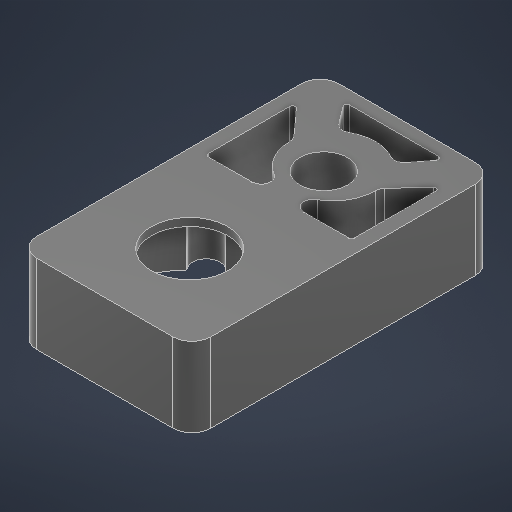
# Autodesk Inventor part: CapOGStyle
Saved by Autodesk Inventor 2026.1 (Build 301233000, 233)
## iProperties
Created: 2023-06-22
Part Number: CapOGStyle
Material: Plastic, Opaque Black
Document SubType Name: Modeling
Designer: Teddy
Density: 0.952 g/cm^3
Appearance: Smooth - Black
Author: Teddy
Autodesk Inventor part; units mm, degrees
ref_plane "YZ Plane" through (0, 0, 0) normal (1, 0, 0) x (0, 1, 0)
ref_plane "XZ Plane" through (0, 0, 0) normal (0, 1, 0) x (-1, 0, 0)
ref_plane "XY Plane" through (0, 0, 0) normal (0, 0, 1) x (1, 0, 0)
sketch "Sketch5" plane through (0, 0, 0) normal (0, 1, 0) x (-1, 0, 0)
  line L0 (-12.8932, 28.65) -> (12.9, 28.65)
  line L1 (16.5, 25.05) -> (16.5, -25.0432)
  line L2 (12.8932, -28.65) -> (-12.8932, -28.65)
  line L3 (-16.5, -25.0432) -> (-16.5, 25.0432)
  line L4 (-16.5, 28.65) -> (16.5, -28.65) construction
  line L5 (16.5, 28.65) -> (-16.5, -28.65) construction
  arc A0 (16.5, 25.05) -> (12.9, 28.65) centre (12.9, 25.05) ccw
  line L6 (12.9, 28.65) -> (12.9, 25.05) construction
  line L7 (12.9, 25.05) -> (16.5, 25.05) construction
  arc A1 (12.8932, -28.65) -> (16.5, -25.0432) centre (12.8932, -25.0432) ccw
  arc A2 (-12.8932, 28.65) -> (-16.5, 25.0432) centre (-12.8932, 25.0432) ccw
  arc A3 (-16.5, -25.0432) -> (-12.8932, -28.65) centre (-12.8932, -25.0432) ccw
  circle A4 centre (13.5, 25.6528) radius 0.9915
  line L8 (11.2085, 27.55) -> (-11.2085, 27.55)
  arc A5 (-15.517, 25.05) -> (-15.517, 25.0432) centre (-12.8932, 25.0432) ccw
  line L9 (-15.4, 23.3613) -> (-15.4, -23.3613)
  line L10 (-11.2085, -27.55) -> (11.2085, -27.55)
  line L11 (15.4, -23.3613) -> (15.4, 23.3613)
  line L12 (12.5085, 25.6528) -> (12.5085, 26.25)
  line L13 (13.5, 24.6613) -> (14.1, 24.6613)
  arc A6 (12.5085, 26.25) -> (11.2085, 27.55) centre (11.2085, 26.25) ccw
  arc A7 (15.4, 23.3613) -> (14.1, 24.6613) centre (14.1, 23.3613) ccw
  line L14 (15.4, 0) -> (-15.4, 0) construction
  line L15 (0, 27.55) -> (0, -27.55) construction
  circle A8 centre (13.5, -25.6528) radius 0.9915
  line L16 (12.5085, -25.6528) -> (12.5085, -26.25)
  line L17 (13.5, -24.6613) -> (14.1, -24.6613)
  arc A9 (11.2085, -27.55) -> (12.5085, -26.25) centre (11.2085, -26.25) ccw
  arc A10 (14.1, -24.6613) -> (15.4, -23.3613) centre (14.1, -23.3613) ccw
  line L18 (0, -27.55) -> (0, 27.55) construction
  circle A11 centre (-13.5, 25.6528) radius 0.9915
  line L19 (-12.5085, 25.6528) -> (-12.5085, 26.25)
  line L20 (-13.5, 24.6613) -> (-14.1, 24.6613)
  arc A12 (-11.2085, 27.55) -> (-12.5085, 26.25) centre (-11.2085, 26.25) ccw
  arc A13 (-14.1, 24.6613) -> (-15.4, 23.3613) centre (-14.1, 23.3613) ccw
  arc A14 (-12.5085, -26.25) -> (-11.2085, -27.55) centre (-11.2085, -26.25) ccw
  line L21 (-12.5085, -25.6528) -> (-12.5085, -26.25)
  circle A15 centre (-13.5, -25.6528) radius 0.9915
  line L22 (-13.5, -24.6613) -> (-14.1, -24.6613)
  arc A16 (-15.4, -23.3613) -> (-14.1, -24.6613) centre (-14.1, -23.3613) ccw
  line L23 (-12.1355, -25.3386) -> (-12.1355, -25.333)
  line L24 (14.7139, 22.2154) -> (14.827, 22.0092) construction
  circle A17 centre (0, 12.583) radius 7.25
  arc A18 (6.3593, 25.2794) -> (-6.3593, 25.2794) centre (0, 12.583) ccw
  arc A19 (-6.3593, -0.1134) -> (6.3593, -0.1134) centre (0, 12.583) ccw
  line L25 (0, 12.583) -> (-6.3593, -0.1134) construction
  line L26 (0, 12.583) -> (6.3593, -0.1134) construction
  line L27 (0, 12.583) -> (0, -1.617) construction
  line L28 (0, 12.583) -> (16.5, 12.583) construction
  line L29 (-6.3593, -0.1134) -> (-6.3593, 25.2794) construction
  line L30 (6.3593, -0.1134) -> (6.3593, 25.2794) construction
  arc A20 (-6.3593, -0.1134) -> (-6.9877, -0.2666) centre (-6.5832, -0.5605) ccw
  line L31 (-6.9877, -0.2666) -> (-6.5832, -0.5605) construction
  line L32 (-6.5832, -0.5605) -> (-6.3593, -0.1134) construction
  line L33 (-6.9877, -0.2666) -> (-7.2816, -0.671)
  arc A21 (-10.5175, 1.6804) -> (-7.2816, -0.671) centre (-8.8995, 0.5047) ccw
  line L34 (-10.5175, 1.6804) -> (-10.2236, 2.0849)
  arc A22 (-10.2236, 2.0849) -> (-10.2728, 2.7402) centre (-10.6345, 2.3835) ccw
  line L35 (-10.2236, 2.0849) -> (-10.6345, 2.3835) construction
  line L36 (-10.6345, 2.3835) -> (-10.2728, 2.7402) construction
  arc A23 (6.9877, -0.2666) -> (6.3593, -0.1134) centre (6.5832, -0.5605) ccw
  line L37 (6.9877, -0.2666) -> (7.2816, -0.671)
  arc A24 (7.2816, -0.671) -> (10.5175, 1.6804) centre (8.8995, 0.5047) ccw
  line L38 (10.5175, 1.6804) -> (10.2236, 2.0849)
  arc A25 (10.2728, 2.7402) -> (10.2236, 2.0849) centre (10.6345, 2.3835) ccw
  arc A26 (-6.9877, 25.4326) -> (-6.3593, 25.2794) centre (-6.5832, 25.7265) ccw
  line L39 (-6.9877, 25.4326) -> (-7.2816, 25.837)
  arc A27 (-7.2816, 25.837) -> (-10.5175, 23.4856) centre (-8.8995, 24.6613) ccw
  line L40 (-10.5175, 23.4856) -> (-10.2236, 23.0811)
  arc A28 (-10.2728, 22.4258) -> (-10.2236, 23.0811) centre (-10.6345, 22.7825) ccw
  arc A29 (6.3593, 25.2794) -> (6.9877, 25.4326) centre (6.5832, 25.7265) ccw
  line L41 (6.9877, 25.4326) -> (7.2816, 25.837)
  arc A30 (10.5175, 23.4856) -> (7.2816, 25.837) centre (8.8995, 24.6613) ccw
  line L42 (10.5175, 23.4856) -> (10.2236, 23.0811)
  arc A31 (10.2236, 23.0811) -> (10.2728, 22.4258) centre (10.6345, 22.7825) ccw
  arc A32 (-10.2728, 22.4258) -> (-10.2728, 2.7402) centre (0, 12.583) ccw
  arc A33 (10.2728, 2.7402) -> (10.2728, 22.4258) centre (0, 12.583) ccw
  circle A34 centre (0, -12.96) radius 3.955
  line L43 (0, -12.96) -> (0, -18.96) construction
  circle A35 centre (13.5, -25.6528) radius 2
  line L44 (13.5, -25.6528) -> (13.5, -23.6528) construction
  line L45 (13.5, -25.6528) -> (11.5, -25.6528) construction
  line L46 (13.5, -23.6528) -> (15.3669, -23.6528) construction
  line L47 (11.5, -25.6528) -> (11.5, -27.5169) construction
  circle A36 centre (-13.5, -25.6528) radius 2
  circle A37 centre (-13.5, 25.6528) radius 2
  circle A38 centre (13.5, 25.6528) radius 2
  circle A39 centre (0, -12.843) radius 4.5212
  circle A40 centre (0, -14.56) radius 6.25
  line L48 (0, -14.56) -> (-5.807, -24.618) construction
  line L49 (0, -14.56) -> (5.807, -24.618) construction
  arc A41 (-4.057, -21.5869) -> (4.057, -21.5869) centre (0, -14.56) ccw
  arc A42 (-4.057, -21.5869) -> (-6.3593, -22.0899) centre (-4.932, -23.1025) ccw
  arc A43 (6.3306, -22.0506) -> (4.057, -21.5869) centre (4.932, -23.1025) ccw
  line L50 (0, -26.174) -> (-8.43, -26.174)
  line L51 (0, -26.174) -> (8.4301, -26.174)
  line L52 (8.8297, -25.3735) -> (6.3306, -22.0506)
  arc A44 (8.4301, -26.174) -> (8.8297, -25.3735) centre (8.4301, -25.674) ccw
  line L53 (-8.8295, -25.3734) -> (-6.3593, -22.0899)
  arc A45 (-8.8295, -25.3734) -> (-8.43, -26.174) centre (-8.43, -25.674) ccw
  line L54 (-4.8269, -4.2707) -> (-13.3585, -4.2707)
  line L55 (-13.8585, -4.7707) -> (-13.8585, -20.2911)
  line L56 (-12.9875, -20.6263) -> (-8.5656, -15.7334)
  arc A46 (-13.8585, -20.2911) -> (-12.9875, -20.6263) centre (-13.3585, -20.2911) ccw
  arc A47 (-13.3585, -4.2707) -> (-13.8585, -4.7707) centre (-13.3585, -4.7707) ccw
  line L57 (5.0371, -4.2707) -> (13.3585, -4.2707)
  line L58 (13.8585, -4.7707) -> (13.8585, -20.2921)
  line L59 (12.9875, -20.6273) -> (8.5655, -15.7332)
  arc A48 (12.9875, -20.6273) -> (13.8585, -20.2921) centre (13.3585, -20.2921) ccw
  arc A49 (13.8585, -4.7707) -> (13.3585, -4.2707) centre (13.3585, -4.7707) ccw
  arc A50 (8.114, -14.56) -> (4.057, -7.5331) centre (0, -14.56) ccw
  arc A51 (-4.057, -7.5331) -> (-8.114, -14.56) centre (0, -14.56) ccw
  arc A52 (8.114, -14.56) -> (8.5655, -15.7332) centre (9.864, -14.56) ccw
  arc A53 (5.0371, -4.2707) -> (4.057, -7.5331) centre (5.0371, -6.0491) ccw
  arc A54 (-4.057, -7.5331) -> (-4.8269, -4.2707) centre (-4.8269, -5.9927) ccw
  arc A55 (-8.5656, -15.7334) -> (-8.114, -14.56) centre (-9.864, -14.56) ccw
  line L60 (10.7841, 22.7925) -> (11.0216, 23.1193)
  arc A56 (11.0216, 23.1193) -> (6.7775, 26.2034) centre (8.8995, 24.6613) ccw
  line L61 (6.7775, 26.2034) -> (6.5448, 25.883)
  arc A57 (6.5448, 25.883) -> (-6.5448, 25.883) centre (0, 12.583) ccw
  line L62 (-6.5448, 25.883) -> (-6.7775, 26.2034)
  arc A58 (-6.7775, 26.2034) -> (-11.0216, 23.1193) centre (-8.8995, 24.6613) ccw
  line L63 (-11.0216, 23.1193) -> (-10.7841, 22.7925)
  arc A59 (-10.7841, 22.7925) -> (-10.7841, 2.3735) centre (0, 12.583) ccw
  line L64 (-10.7841, 2.3735) -> (-11.0216, 2.0467)
  arc A60 (-11.0216, 2.0467) -> (-6.7775, -1.0374) centre (-8.8995, 0.5047) ccw
  line L65 (-6.7775, -1.0374) -> (-6.5448, -0.717)
  arc A61 (-6.5448, -0.717) -> (6.5448, -0.717) centre (0, 12.583) ccw
  line L66 (6.5448, -0.717) -> (6.7775, -1.0374)
  arc A62 (6.7775, -1.0374) -> (11.0216, 2.0467) centre (8.8995, 0.5047) ccw
  line L67 (11.0216, 2.0467) -> (10.7841, 2.3735)
  arc A63 (10.7841, 2.3735) -> (10.7841, 22.7925) centre (0, 12.583) ccw
  point P0 (0, 0)
  point P1 (0, 0)
  point P2 (-2.4, 0)
  point P3 (-12.1591, 27.1367)
  point P4 (-14.9852, 24.3133)
  point P5 (-14.9852, -24.3133)
  point P6 (-12.1591, -27.1367)
  point P7 (12.1591, -27.1367)
  point P8 (14.9852, -24.3133)
  point P9 (14.9852, 24.3133)
  point P10 (12.1591, 27.1367)
  point P11 (5.807, -24.501)
  point P12 (13.8585, -4.2707)
  dimension "d61" = 57.3
  dimension "d62" = 33
  dimension "d63" = 3.6
  dimension "d64" = 90
  dimension "d65" = 3.6068
  dimension "d66" = 3.6068
  dimension "d67" = 2.9972
  dimension "d68" = 3
  dimension "d69" = 1.983
  dimension "d70" = 1.1
  dimension "d71" = 1.3
  dimension "d74" = 22.417
  dimension "d84" = 14.5
  dimension "d85" = 28.4
  dimension "d87" = 53.21
  dimension "d88" = 0.5
  dimension "d89" = 80.6
  dimension "d90" = 0.5
  dimension "d91" = 2
  dimension "d92" = 0.508
  dimension "d93" = 80.6
  dimension "d98" = 25.543
  dimension "d99" = 7.91
  dimension "d116" = 4
  dimension "d117" = 4
  dimension "d118" = 4
  dimension "d119" = 4
  dimension "d128" = 9.0424
  dimension "d129" = 1.6
  dimension "d130" = 12.5
  dimension "d131" = 60
  dimension "d132" = 30
  dimension "d145" = 0.5
  dimension "d146" = 0.5
  dimension "d147" = 0.5
  dimension "d148" = 0.5
  dimension "d151" = 360
  dimension "d192" = 1.1
  dimension "d193" = 1.1
  dimension "d195" = 1.1
  constraints: 136 end point, 120 point on circle, 64 centre point, 53 symmetric about line, 37 tangent, 20 point on line, 11 coincident, 9 perpendicular, 6 midpoint, 5 parallel, 4 equal radius, 4 vertical, 3 horizontal, 1 collinear, 45 other
  measures "d61" distance of L5.start L4.end
  measures "d62" distance of L4.end L5.end
  measures "d63" radius of A0
  measures "d64" angle of L6 L7
  measures "d65" radius of A1
  measures "d66" radius of A2
  measures "d67" distance from line of L0 A4.centre
  measures "d68" distance from line of L1 A4.centre
  measures "d69" diameter of A4
  measures "d70" distance between parallel lines of L0 L8
  measures "d71" radius of A6
  measures "d74" distance of L10.start L10.end
  measures "d84" diameter of A17
  measures "d85" diameter of A18
  measures "d87" angle of L25 L26
  measures "d88" radius of A20
  measures "d89" angle of L32 L31
  measures "d90" distance of L31.start L33.end
  measures "d91" radius of A21
  measures "d92" radius of A22
  measures "d93" angle of L36 L35
  measures "d98" distance of A17.centre A34.centre
  measures "d99" diameter of A34
  measures "d116" diameter of A35
  measures "d117" diameter of A36
  measures "d118" diameter of A37
  measures "d119" diameter of A38
  measures "d128" diameter of A39
  measures "d129" distance of A34.centre L48.start
  measures "d130" diameter of A40
  measures "d131" angle of L49 L48
  measures "d132" angle of L43 L48
  measures "d145" radius of A44
  measures "d146" radius of A45
  measures "d147" radius of A46
  measures "d148" radius of A48
  measures "d192" distance between parallel lines of L3 L9
  measures "d193" distance between parallel lines of L2 L10
  measures "d195" distance between parallel lines of L1 L11
extrude "Extrusion6" add sketch "Sketch5" against normal blind 13.5 contours L0 A0 L1 A1 L2 A3 L3 A2 | A4 | A4 L12 A6 A38 A7 L13 | A4 L13 A7 A38 A6 L12 | A38 A7 L11 A10 A35 A9 L10 A14 A36 A16 L9 A13 A37 A12 L8 A6 | A37 A13 L20 A11 L19 A12 | A12 L19 A11 L20 A13 A37 | A35 A9 L16 A8 L17 A10 | A10 L17 A8 L16 A9 A35 | A11 | A8 | A36 A14 L21 A15 L22 A16 | A16 L22 A15 L21 A14 A36 | A15 | A29 L41 A30 L42 A31 A33 A25 L38 A24 L37 A23 A19 A20 L33 A21 L34 A22 A32 A28 L40 A27 L39 A26 A18 | A34 | A39 | A40 | A41 A43 L52 A44 L51 L50 A45 L53 A42 | A54 A51 A55 L56 A46 L55 A47 L54 | L57 A49 L58 A48 L59 A52 A50 A53 | A63 L67 A62 L66 A61 L65 A60 L64 A59 L63 A58 L62 A57 L61 A56 L60
extrude "Extrusion9" cut sketch "Sketch5" against normal blind 22 contours A4 L13 A7 A38 A6 L12 | A38 A7 L11 A10 A35 A9 L10 A14 A36 A16 L9 A13 A37 A12 L8 A6 | A37 A13 L20 A11 L19 A12 | A10 L17 A8 L16 A9 A35 | A36 A14 L21 A15 L22 A16 | A29 L41 A30 L42 A31 A33 A25 L38 A24 L37 A23 A19 A20 L33 A21 L34 A22 A32 A28 L40 A27 L39 A26 A18 | A34 | A39 | A40 | A41 A43 L52 A44 L51 L50 A45 L53 A42 | A54 A51 A55 L56 A46 L55 A47 L54 | L57 A49 L58 A48 L59 A52 A50 A53 | A63 L67 A62 L66 A61 L65 A60 L64 A59 L63 A58 L62 A57 L61 A56 L60 picked at (13.7589, 24.3277) picked at (-13.7763, 24.3295) picked at (13.7589, -24.3277) picked at (-13.7763, -24.3295)
extrude "Extrusion10" add sketch "Sketch5" against normal blind 12.5 contours A4 L13 A7 A38 A6 L12 | A37 A13 L20 A11 L19 A12 | A10 L17 A8 L16 A9 A35 | A36 A14 L21 A15 L22 A16 picked at (13.7589, 24.3277) picked at (-13.7763, 24.3295) picked at (13.7589, -24.3277) picked at (-13.7763, -24.3295)
extrude "Extrusion11" add sketch "Sketch5" against normal blind 11.5 contours A34 | A39 | A40
extrude "Extrusion12" cut sketch "Sketch5" against normal blind 11.5 contours A34 | A39
extrude "Extrusion13" add sketch "Sketch5" against normal blind 12.5 contours A38 A7 L11 A10 A35 A9 L10 A14 A36 A16 L9 A13 A37 A12 L8 A6
extrude "Extrusion14" add sketch "Sketch5" along normal blind 1.5 contours L0 A0 L1 A1 L2 A3 L3 A2 | A4 | A4 L12 A6 A38 A7 L13 | A4 L13 A7 A38 A6 L12 | A38 A7 L11 A10 A35 A9 L10 A14 A36 A16 L9 A13 A37 A12 L8 A6 | A37 A13 L20 A11 L19 A12 | A12 L19 A11 L20 A13 A37 | A35 A9 L16 A8 L17 A10 | A10 L17 A8 L16 A9 A35 | A11 | A8 | A36 A14 L21 A15 L22 A16 | A16 L22 A15 L21 A14 A36 | A15 | A29 L41 A30 L42 A31 A33 A25 L38 A24 L37 A23 A19 A20 L33 A21 L34 A22 A32 A28 L40 A27 L39 A26 A18 | A40 | A63 L67 A62 L66 A61 L65 A60 L64 A59 L63 A58 L62 A57 L61 A56 L60
sketch "Sketch13" plane through (0, 0, 0) normal (0, -1, 0) x (1, 0, 0)
  arc A0 (-6.5448, -0.717) -> (6.5448, -0.717) centre (0, 12.583) ccw construction
  line L0 (0, -2.2401) -> (0, 1.5699) construction
  arc A1 (1.048, -2.203) -> (-1.048, -2.203) centre (0, -0.4621) ccw
  arc A2 (-1.048, -2.203) -> (1.048, -2.203) centre (0, 12.583) ccw
  line L1 (1.5178, -2.1622) -> (1.8929, -1.2009)
  line L2 (-1.8929, -1.2009) -> (-1.5178, -2.1622)
  arc A3 (-1.5178, -2.1622) -> (1.5178, -2.1622) centre (0, 12.583) ccw
  point P0 (0, 0)
  point P1 (-1.048, -2.203)
  point P2 (1.048, -2.203)
  dimension "d204" = 3.81
  dimension "d205" = 2.032
  constraints: 16 point on circle, 6 end point, 3 centre point, 2 tangent, 1 point on line, 1 vertical
  measures "d204" distance of L0.start L0.end
  measures "d205" radius of A1
extrude "Extrusion22" add sketch "Sketch13" along normal blind 1.5
body "Solid2"
